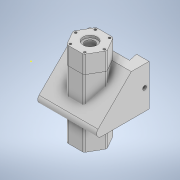
# Autodesk Inventor part: Część8
Saved by Autodesk Inventor 2021 (Build 250183000, 183)
## iProperties
Created: 2023-09-26
Part Number: Część8
Material: Ogólny
Document SubType Name: Modeling
Designer: Jakub
Density: 1 g/cm^3
Appearance: Domyślna
Author: Jakub
Autodesk Inventor part; units mm, degrees
ref_plane "YZ Plane" through (0, 0, 0) normal (1, 0, 0) x (0, 1, 0)
ref_plane "XZ Plane" through (0, 0, 0) normal (0, 1, 0) x (-1, 0, 0)
ref_plane "XY Plane" through (0, 0, 0) normal (0, 0, 1) x (1, 0, 0)
sketch "Szkic1" plane through (0, 0, 0) normal (0, 1, 0) x (-1, 0, 0)
  line L0 (0, 0) -> (-50, 0)
  line L1 (-50, 0) -> (-50, -50)
  line L2 (0, 0) -> (0, -50)
  line L3 (-9, -42.5) -> (-41, -42.5)
  line L4 (-9, -42.5) -> (-10.5942, -50)
  line L5 (-9, -42.5) -> (-1.3324, -42.5) construction
  line L6 (-41, -42.5) -> (-39.4058, -50)
  line L7 (-41, -42.5) -> (-33.3324, -42.5) construction
  line L8 (-39.4058, -50) -> (-50, -50)
  line L9 (-10.5942, -50) -> (0, -50)
  dimension "d0" = 50
  dimension "d1" = 50
  dimension "d26" = 102
  dimension "d27" = 78
  constraints: 20 end point, 5 horizontal, 2 equal length, 1 perpendicular
  measures "d0" distance of L0.start L0.end
  measures "d1" distance of L0.end L1.end
  measures "d26" angle of L4 L5
  measures "d27" angle of L6 L7
extrude "Wyciągnięcie proste1" add sketch "Szkic1" along normal blind 35
chamfer "Faza1" distance 35 angle 45 1 edges at (25, 35, 0) measured on face at (25, 35, -0.5)
fillet "Zaokrąglenie1" radius 4 4 edges at (50, 0.0001, 0) (0, 0.0001, 0) (25, 0.0001, 0) (25, 0, 0)
sketch "Szkic5" plane through (0, 35, 0) normal (0, 1, 0) x (1, 0, 0)
  line L0 (50, 50) -> (0, 50) projected
  line L1 (25, 50) -> (25, 25)
  line L2 (25, 25) -> (50, 25)
  line L3 (50, 9.6569) -> (50, 50) projected
  line L4 (25, 25) -> (25, 37.5)
  line L5 (27.4454, 25) -> (27.4454, 37.5)
  line L6 (17.7996, 37.5) -> (32.2251, 37.4857)
  line L7 (32.2251, 37.4857) -> (39.4255, 24.9857)
  line L8 (39.4255, 24.9857) -> (32.2004, 12.5)
  line L9 (32.2004, 12.5) -> (17.7749, 12.5143)
  line L10 (17.7749, 12.5143) -> (10.5745, 25.0143)
  line L11 (10.5745, 25.0143) -> (17.7996, 37.5)
  point P0 (0, 0)
  dimension "d10" = 25
  dimension "d11" = 12.5
  constraints: 20 end point, 2 midpoint, 2 point on line, 2 vertical, 1 coincident, 1 perpendicular, 13 other
  measures "d10" distance of L1.start L1.end
  measures "d11" distance of L5.start L5.end
sketch "Szkic6" plane through (0, 35, 0) normal (0, 1, 0) x (1, 0, 0)
  point P0 (0, 0)
extrude "Wyciągnięcie proste2" add sketch "Szkic5" against normal blind 57 separate body contours L7 L8 L9 L10 L11 L6 L1 L2 | L2 L5 L6 L7 | L6 L5 L2 L1
sketch "Szkic7" plane through (0, 35, 0) normal (0, 1, 0) x (1, 0, 0)
  line L0 (17.7749, 12.5143) -> (10.5745, 25.0143) projected
  line L1 (32.2251, 37.4857) -> (39.4255, 24.9857) projected
  line L2 (10.5745, 25.0143) -> (39.4255, 24.9857)
  line L3 (39.4255, 24.9857) -> (25, 25)
  line L4 (17.7996, 37.5) -> (32.2251, 37.4857) projected
  line L5 (32.2251, 37.4857) -> (39.4255, 24.9857)
  line L6 (39.4255, 24.9857) -> (32.2004, 12.5)
  line L7 (32.2004, 12.5) -> (17.7749, 12.5143)
  line L8 (17.7749, 12.5143) -> (10.5745, 25.0143)
  line L9 (10.5745, 25.0143) -> (17.7996, 37.5)
  line L10 (17.7996, 37.5) -> (32.2251, 37.4857)
  point P0 (0, 0)
  constraints: 16 end point, 1 coincident, 1 midpoint, 13 other
extrude "Wyciągnięcie proste3" add sketch "Szkic7" along normal blind 15 separate body
fillet "Zaokrąglenie2" radius 2 1 edges at (17.7996, 42.5, -37.5)
fillet "Zaokrąglenie3" radius 2 1 edges at (32.2251, 42.5, -37.4857)
fillet "Zaokrąglenie4" radius 2 1 edges at (39.4255, 42.5, -24.9857)
fillet "Zaokrąglenie5" radius 2 1 edges at (32.2004, 42.5, -12.5)
fillet "Zaokrąglenie6" radius 2 1 edges at (17.7749, 42.5, -12.5143)
fillet "Zaokrąglenie7" radius 2 1 edges at (10.5745, 42.5, -25.0143)
fillet "Zaokrąglenie8" radius 2 6 edges at (10.5745, 6.5, -25.0143) (17.7749, 6.5, -12.5143) (32.2004, 6.5, -12.5) (39.4255, 6.5, -24.9857) (32.2251, 6.5, -37.4857) (17.7996, 6.5, -37.5)
sketch "Szkic8" plane through (0, 0, -50) normal (-1, 0, 0) x (0, 0, 1)
  line L0 (7.5, 35) -> (0, 35) projected
  line L1 (0, 35) -> (0, 17.5)
  line L2 (0, 0) -> (0, 35) projected
  line L3 (0, 17.5) -> (3.75, 17.5)
  point P0 (50, 0)
  constraints: 4 end point, 1 horizontal, 1 midpoint
hole "Otwór1" at (0, 17.5, -46.25) direction (1, 0, 0) diameter 3.242 end through all bodies 1 thread size "M4x0.7" class "6H" standard "ANSI Metric M Profile"
sketch "Szkic9" plane through (0, 50, 0) normal (0, 1, 0) x (1, 0, 0)
  arc A0 (18.9543, 37.4989) -> (17.2213, 36.5006) centre (18.9524, 35.4989) ccw projected
  arc A1 (32.8015, 36.4851) -> (31.0704, 37.4868) centre (31.0685, 35.4868) ccw projected
  line L0 (18.9524, 35.4989) -> (31.0685, 35.4868)
  arc A2 (31.0457, 12.5011) -> (32.7787, 13.4994) centre (31.0476, 14.5011) ccw projected
  line L1 (31.0685, 35.4868) -> (31.0476, 14.5011)
  arc A3 (17.1985, 13.5149) -> (18.9296, 12.5132) centre (18.9315, 14.5132) ccw projected
  line L2 (31.0476, 14.5011) -> (18.9315, 14.5132)
  line L3 (18.9315, 14.5132) -> (18.9524, 35.4989)
  arc A4 (11.1528, 26.0137) -> (11.1509, 24.0137) centre (12.8839, 25.012) ccw projected
  arc A5 (38.8472, 23.9863) -> (38.8491, 25.9863) centre (37.1161, 24.988) ccw projected
  line L4 (12.8839, 25.012) -> (37.1161, 24.988)
  point P0 (0, 0)
  constraints: 10 end point, 3 perpendicular
hole "Otwór2" at (12.8839, 50, -25.012) at (18.9524, 50, -35.4989) at (31.0685, 50, -35.4868) at (37.1161, 50, -24.988) at (31.0476, 50, -14.5011) at (18.9315, 50, -14.5132) direction (0, -1, 0) diameter 1.8129 depth 4 bodies 3 thread size "M2.3x0.45" class "6H" standard "ANSI Metric M Profile"
sketch "Szkic10" plane through (0, 50, 0) normal (0, 1, 0) x (1, 0, 0)
  circle A0 centre (12.8839, 25.012) radius 0.9064 projected
  line L0 (12.8839, 25.012) -> (37.2382, 25.012)
  line L1 (37.2382, 25.012) -> (25, 35)
  line L2 (50, 35) -> (0, 35) projected
  line L3 (25, 35) -> (25.0611, 25.012)
  circle A1 centre (25.0611, 25.012) radius 6
  point P0 (0, 0)
  dimension "d42" = 12
  constraints: 6 end point, 2 midpoint, 1 centre point, 1 coincident, 1 horizontal
  measures "d42" diameter of A1
extrude "Wyciągnięcie proste4" cut sketch "Szkic10" against normal blind 2 contours L3 A1 L0 | L0 A1 | L0 A1 L3 bodies 3
sketch "Szkic11" plane through (0, 50, 0) normal (0, 1, 0) x (1, 0, 0)
  circle A0 centre (25, 25) radius 4
  point P0 (0, 0)
  dimension "d45" = 8
  constraints: 1 centre point
  measures "d45" diameter of A0
hole "Otwór3" at (25, 50, -25) direction (0, -1, 0) diameter 8 depth 100 bodies 3 1 2
